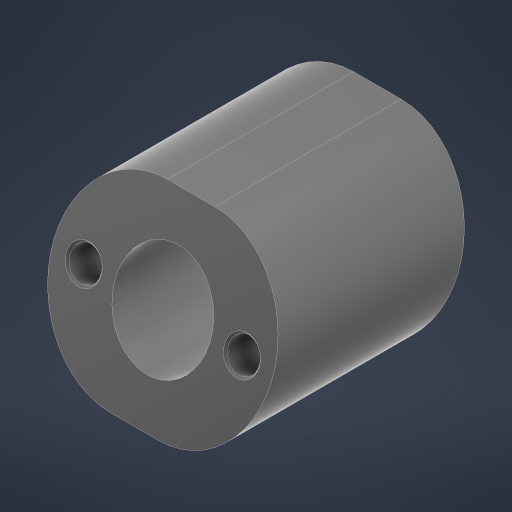
# Autodesk Inventor part: Leg_Loadpipe_Mount
Saved by Autodesk Inventor 2024 (Build 280153000, 153)
## iProperties
Created: 2023-06-09
Part Number: Leg_Loadpipe_Mount
Material: Nylon 6/6
Document SubType Name: Modeling
Designer: dzw04
Density: 1.13 g/cm^3
Appearance: Smooth - Black
Author: dzw04
Autodesk Inventor part; units mm, degrees
ref_plane "YZ Plane" through (0, 0, 0) normal (1, 0, 0) x (0, 1, 0)
ref_plane "XZ Plane" through (0, 0, 0) normal (0, 1, 0) x (-1, 0, 0)
ref_plane "XY Plane" through (0, 0, 0) normal (0, 0, 1) x (1, 0, 0)
sketch "Sketch1" plane through (0, 0, 0) normal (1, 0, 0) x (0, 1, 0)
  line L0 (0, 0) -> (35.6646, -11.5881) construction
  line L1 (0, 0) -> (37.5, 0) construction
  line L2 (35.6646, -11.5881) -> (35.0466, -13.4903) construction
  line L3 (35.0466, -13.4903) -> (-0.618, -1.9021) construction
  line L4 (-0.618, -1.9021) -> (0, 0) construction
  line L5 (35.0466, -13.4903) -> (28.1246, -34.7939) construction
  line L6 (28.1246, -34.7939) -> (-7.54, -23.2058) construction
  line L7 (-7.54, -23.2058) -> (-8.158, -25.1079) construction
  line L8 (-8.158, -25.1079) -> (27.5066, -36.696) construction
  line L9 (27.5066, -36.696) -> (28.1246, -34.7939) construction
  line L10 (17.2143, -7.6962) -> (9.6743, -28.799) construction
  line L11 (13.4443, 23.5996) -> (13.4443, -60.0949) construction
  line L12 (7.4443, 23.5996) -> (7.4443, -60.0949) construction
  line L13 (19.4443, 23.5996) -> (19.4443, -60.0949) construction
  line L14 (13.4443, -4.3683) -> (24.3814, -7.922) construction
  line L15 (24.3814, -7.922) -> (16.2234, -33.0299) construction
  line L16 (13.4443, -4.3683) -> (2.5071, -0.8146) construction
  line L17 (2.5071, -0.8146) -> (-5.6509, -25.9225) construction
  line L18 (2.4443, 23.5996) -> (2.4443, -60.0949)
  line L19 (24.4443, 23.5996) -> (24.4443, -60.0949)
  line L20 (19.5693, 23.5996) -> (19.5693, -60.0949)
  line L21 (7.3193, 23.5996) -> (7.3193, -60.0949)
  line L22 (2.4443, -2.8971) -> (7.3193, -4.4811)
  line L23 (2.4443, -26.4499) -> (7.3193, -28.0339)
  line L24 (24.4443, -33.5981) -> (19.5693, -32.0141)
  line L25 (24.4443, -10.0453) -> (19.5693, -8.4614)
  point P0 (13.4443, -18.2476)
  dimension "d1" = 37.5
  dimension "d2" = 18
  dimension "d3" = 2
  dimension "d4" = 22.4
  dimension "d5" = 37.5
  dimension "d6" = 2
  dimension "d7" = 6
  dimension "d8" = 6
  dimension "d9" = 11.5
  dimension "d10" = 11.5
  dimension "d13" = 11
  dimension "d14" = 11
  dimension "d15" = 4.875
  dimension "d16" = 4.875
  constraints: 52 end point, 24 point on line, 9 perpendicular, 6 parallel, 3 midpoint, 1 equal length, 1 horizontal, 1 vertical
  measures "d1" distance of L0.start L0.end
  measures "d2" angle of L0 L1
  measures "d3" distance of L0.end L2.end
  measures "d4" distance of L2.end L5.end
  measures "d5" distance of L5.end L6.end
  measures "d6" distance of L6.end L7.end
  measures "d7" distance between parallel lines of L11 L12
  measures "d8" distance between parallel lines of L13 L11
  measures "d9" distance of L14.start L14.end
  measures "d10" distance of L14.start L16.end
  measures "d13" distance between parallel lines of L11 L18
  measures "d14" distance between parallel lines of L11 L19
  measures "d15" distance between parallel lines of L19 L20
  measures "d16" distance between parallel lines of L18 L21
extrude "Extrusion1" add sketch "Sketch1" along normal blind 28
sketch "Sketch2" plane through (28, 0, 0) normal (1, 0, 0) x (0, 0, -1)
  line L0 (28.0339, 7.3193) -> (4.4811, 7.3193) projected
  line L1 (8.4614, 19.5693) -> (32.0141, 19.5693) projected
  line L2 (4.4811, 7.3193) -> (8.4614, 19.5693)
  line L3 (8.4614, 19.5693) -> (32.0141, 19.5693)
  line L4 (32.0141, 19.5693) -> (28.0339, 7.3193)
  line L5 (28.0339, 7.3193) -> (4.4811, 7.3193)
  point P0 (0, 0)
  constraints: 8 end point, 3 equal length
extrude "Extrusion2" add sketch "Sketch2" against normal blind 7.875
sketch "Sketch3" plane through (0, 0, 0) normal (-1, 0, 0) x (0, 0, 1)
  line L0 (-8.4614, 19.5693) -> (-32.0141, 19.5693) projected
  line L1 (-26.4499, 2.4443) -> (-28.0339, 7.3193) projected
  line L2 (-32.0141, 19.5693) -> (-28.0339, 7.3193)
  line L3 (-28.0339, 7.3193) -> (-4.4811, 7.3193)
  line L4 (-4.4811, 7.3193) -> (-8.4614, 19.5693)
  line L5 (-8.4614, 19.5693) -> (-32.0141, 19.5693)
  point P0 (0, 0)
  constraints: 8 end point, 2 parallel, 1 collinear
extrude "Extrusion3" add sketch "Sketch3" against normal blind 7.875
fillet "Fillet1" radius 6.125 4 edges at (7.875, 7.3193, -16.2575) (20.125, 7.3193, -16.2575) (20.125, 19.5693, -20.2377) (7.875, 19.5693, -20.2377)
fillet "Fillet2" radius 11 4 edges at (0, 24.4443, -21.8217) (0, 2.4443, -14.6735) (28, 2.4443, -14.6735) (28, 24.4443, -21.8217)
sketch "Sketch4" plane through (11, 24.4443, -10.0453) normal (0, 0.309017, 0.9510565) x (1, 0, 0)
  ellipse E0 centre (3, -11.5661) end of major axis (3, -18.0063) minor radius 6.125 construction
  circle A0 centre (3, -11.5661) radius 10 construction
  circle A1 centre (-7, -11.5661) radius 2
  circle A2 centre (13, -11.5661) radius 2
  point P0 (-11, -26.3521)
  dimension "d25" = 20
  dimension "d26" = 4
  dimension "d27" = 4
  constraints: 3 centre point, 2 point on circle, 1 coincident, 1 other
  measures "d25" diameter of A0
  measures "d26" diameter of A1
  measures "d27" diameter of A2
extrude "Extrusion4" cut sketch "Sketch4" against normal blind 8
sketch "Sketch5" plane through (17, 2.4443, -26.4499) normal (0, -0.309017, -0.9510565) x (-1, 0, 0)
  ellipse E0 centre (3, 11.5661) end of major axis (3, 18.0063) minor radius 6.125 projected
  circle A0 centre (3, 11.5661) radius 10 construction
  circle A1 centre (-7, 11.5661) radius 2
  circle A2 centre (13, 11.5661) radius 2
  point P0 (17, -10.4981)
  dimension "d30" = 20
  dimension "d31" = 4
  dimension "d32" = 4
  constraints: 3 centre point, 2 point on circle, 1 coincident, 1 other
  measures "d30" diameter of A0
  measures "d31" diameter of A1
  measures "d32" diameter of A2
extrude "Extrusion5" cut sketch "Sketch5" against normal blind 8 contours A1 | A2
sketch "Sketch6" plane through (11, 2.4443, -2.8971) normal (0, -1, 0) x (1, 0, 0)
  line L0 (0, -23.5528) -> (0, 0) projected
  line L1 (0, -11.7764) -> (6, -11.7764) construction
  line L2 (6, 0) -> (6, -23.5528) projected
  circle A0 centre (3, -11.7764) radius 2
  point P0 (-11, 2.8971)
  dimension "d35" = 4
  constraints: 3 midpoint, 2 end point, 1 centre point
  measures "d35" diameter of A0
extrude "Extrusion6" cut sketch "Sketch6" against normal blind 4.25
chamfer "Chamfer1" distance 0.25 angle 45 5 edges at (12, 2.4443, -14.6735) (6, 13.4443, -30.024) (26, 13.4443, -30.024) (22, 13.4443, -6.4712) (2, 13.4443, -6.4712)
body "Solid1"
